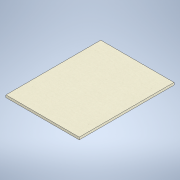
# Autodesk Inventor part: Rules
Saved by Autodesk Inventor 2021 (Build 250183000, 183)
## iProperties
Created: 2023-03-16
Part Number: Rules
Material: Paper
Document SubType Name: Modeling
Designer: Bradley
Density: 0.93 g/cm^3
Appearance: Cardboard - Chipboard
Author: Bradley
Autodesk Inventor part; units mm, degrees
ref_plane "YZ Plane" through (0, 0, 0) normal (1, 0, 0) x (0, 1, 0)
ref_plane "XZ Plane" through (0, 0, 0) normal (0, 1, 0) x (-1, 0, 0)
ref_plane "XY Plane" through (0, 0, 0) normal (0, 0, 1) x (1, 0, 0)
sketch "Sketch1" plane through (0, 0, 0) normal (0, 1, 0) x (-1, 0, 0)
  line L0 (107.95, 139.7) -> (-107.95, 139.7)
  line L1 (-107.95, 139.7) -> (-107.95, -139.7)
  line L2 (-107.95, -139.7) -> (107.95, -139.7)
  line L3 (107.95, -139.7) -> (107.95, 139.7)
  line L4 (107.95, 139.7) -> (-107.95, -139.7) construction
  line L5 (-107.95, 139.7) -> (107.95, -139.7) construction
  point P0 (0, 0)
  dimension "d0" = 215.9
  dimension "d1" = 279.4
  constraints: 12 end point, 2 midpoint, 2 parallel, 1 horizontal, 1 perpendicular
  measures "d0" distance of L2.end L1.end
  measures "d1" distance of L1.end L0.end
extrude "Extrusion1" add sketch "Sketch1" along normal mid plane 7
body "Solid1"
